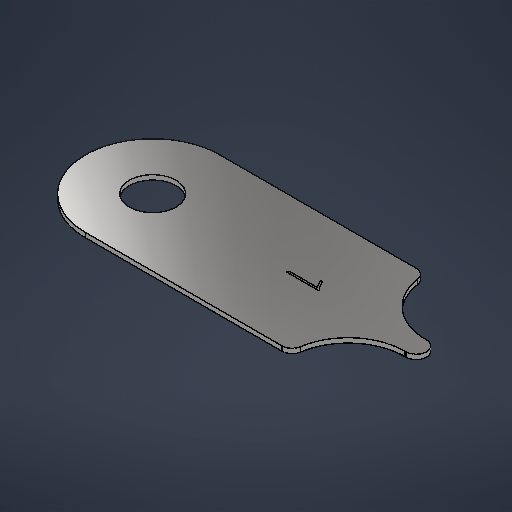
# Autodesk Inventor part: Part16.5mm
Saved by Autodesk Inventor 2026 (Build 300175050, 175E)
## iProperties
Created: 2025-07-21
Part Number: Part16.5mm
Material: Steel, Carbon
Document SubType Name: Sheet Metal
Designer: Joshua Eah
Density: 7.85 g/cm^3
Sheet Metal Rule: 0.4mm Spring Steel
Appearance: Semi-Polished
Author: Joshua Eah
Autodesk Inventor part; units mm, degrees
note: some values were not read from the file. Chosen so that the rebuilt part matches the saved one: direction of "Emboss2".
ref_plane "YZ Plane" through (0, 0, 0) normal (1, 0, 0) x (0, 1, 0)
ref_plane "XZ Plane" through (0, 0, 0) normal (0, 1, 0) x (-1, 0, 0)
ref_plane "XY Plane" through (0, 0, 0) normal (0, 0, 1) x (1, 0, 0)
sketch "Sketch1" plane through (0, 0, 0) normal (0, 1, 0) x (-1, 0, 0)
  line L0 (0, 0) -> (-33, 0) construction
  line L1 (-6.5, 6.5) -> (-26.5, 6.5)
  line L2 (-26.5, -6.5) -> (-6.5, -6.5)
  arc A0 (-6.5, -6.5) -> (-6.5, 6.5) centre (-6.5, 0) ccw
  arc A1 (-26.5, 6.5) -> (-26.5, -6.5) centre (-26.5, 0) ccw
  circle A2 centre (-6.5, 0) radius 2
  line L3 (-22.6527, -1.0329) -> (-22.6527, 4.8111) construction
  line L4 (-22.6527, 4.8111) -> (-19.4837, 4.8111) construction
  line L5 (-19.4837, 4.8111) -> (-19.4837, -1.0329) construction
  line L6 (-19.4837, -1.0329) -> (-22.6527, -1.0329) construction
  line L7 (-26.5, 0) -> (-33, 0) construction
  line L8 (-26.5, -6.5) -> (-26.5, 6.5)
  line L9 (-33, 0) -> (-16.5, 0) construction
  line L10 (-32, -1) -> (-17.5, -1)
  line L11 (-17.5, 1) -> (-32, 1)
  arc A3 (-32, 1) -> (-32, -1) centre (-32, 0) ccw
  arc A4 (-17.5, -1) -> (-17.5, 1) centre (-17.5, 0) ccw
  line L12 (-22.6527, 0.0867) -> (-19.5369, 0.0867)
  line L13 (-19.5369, 0.0867) -> (-19.5369, -0.1112)
  line L14 (-19.5369, -0.1112) -> (-22.3445, -0.1112)
  spline S0 degree 2 poles (-22.3445, -0.1112) (-22.2032, -0.2582) (-21.9996, -0.6343) (-21.9204, -0.8576) knots 0 0 0 1 2 2 2
  line L15 (-21.9204, -0.8576) -> (-22.0985, -0.8576)
  spline S1 degree 2 poles (-22.0985, -0.8576) (-22.1438, -0.7219) (-22.2569, -0.4929) (-22.3926, -0.2836) (-22.5566, -0.0857) (-22.6527, 0.0161) knots 0 0 0 1 2 3 4 4 4
  line L16 (-22.6527, 0.0161) -> (-22.6527, 0.0867)
  point P0 (-29.75, 0)
  point P1 (-24.75, 0)
  point P2 (-26.5, -1)
  point P3 (-26.5, 1)
  dimension "d0" = 33
  dimension "d1" = 13
  dimension "d2" = 4
  dimension "d18" = 2
  dimension "d19" = 5.5
  constraints: 22 end point, 12 point on circle, 8 tangent, 5 centre point, 4 point on line, 3 midpoint, 2 collinear, 2 parallel, 1 coincident, 1 horizontal, 1 vertical, 3 other
  measures "d0" distance of L0.start L0.end
  measures "d1" diameter of A1
  measures "d2" diameter of A2
  measures "d18" diameter of A4
  measures "d19" distance from line of L1.end L11
extrude "Plate1" add sketch "Sketch1" against normal blind 0.45 contours A0 L2 L8 L10 A4 L11 L1 | A3 L11 L8 L10 | L11 A4 L10 L8 | A2 | L12 L13 L14 S0 L15 S1 L16
hole "Hole1" at (6.5, 0, 0) direction (0, -1, 0) diameter 4.4958 end through all clearance for "Socket Head Cap Screw" size "M4" standard "Ansi Metric M Profile"
emboss "Emboss2" sketch "Sketch1" operation cut depth 0.01 direction (0, -1, 0) draft 45 contours L12 L13 L14 S0 L15 S1 L16
fillet "Fillet1" radius 1 2 edges at (26.5, -0.225, 6.5) (26.5, -0.225, -6.5)
fillet "Fillet3" radius 5.5 2 edges at (26.5, -0.225, 1) (26.5, -0.225, -1)
equation "\"d9\" = Thickness"
equation "\"d20\" = d19"
equation "\"d3\" = Thickness"
equation "\"BendRadius\" = Thickness"
equation "\"BendReliefWidth\" = Thickness"
equation "\"BendReliefDepth\" = 0.5 * Thickness"
equation "\"CornerReliefSize\" = 4 * Thickness"
equation "\"MinimumRemnant\" = 2 * Thickness"
equation "\"TransitionRadius\" = BendRadius"
equation "\"JacobiRadiusSize\" = BendRadius"
equation "\"GapSize\" = Thickness"
equation "\"Thickness\" = 0.45"
body "Solid1"
